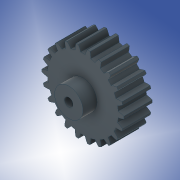
# Autodesk Inventor part: BA011
Saved by Autodesk Inventor 2017 (Build 210142000, 142)
## iProperties
Created: 2017-06-23
Part Number: BA011
Material: ABS Plastic
Document SubType Name: Modeling
Designer: zallen
Density: 1.06 g/cm^3
Appearance: CR Dark Blue
Author: zallen
Autodesk Inventor part; units mm, degrees
ref_plane "YZ Plane" through (0, 0, 0) normal (1, 0, 0) x (0, 1, 0)
ref_plane "XZ Plane" through (0, 0, 0) normal (0, 1, 0) x (-1, 0, 0)
ref_plane "XY Plane" through (0, 0, 0) normal (0, 0, 1) x (1, 0, 0)
sketch "Sketch1" plane through (0, 0, 0) normal (0, 0, 1) x (1, 0, 0)
  circle A0 centre (0, 0) radius 3
  circle A1 centre (0, 0) radius 25
  dimension "d0" = 6
  dimension "d1" = 50
  constraints: 2 centre point, 2 coincident
  measures "d0" diameter of A0
  measures "d1" diameter of A1
extrude "Extrusion1" add sketch "Sketch1" along normal blind 20
sketch "Sketch2" plane through (0, 0, 20) normal (0, 0, 1) x (1, 0, 0)
  line L0 (0, 0) -> (50, 0) construction
  circle A0 centre (0, 0) radius 25 projected
  circle A1 centre (0, 0) radius 25 projected
  arc A2 (28.9199, 0.9) -> (24.9199, 2) centre (22.9807, -12.8741) ccw
  arc A3 (28.9199, -0.9) -> (28.9199, 0.9) centre (8.9401, 0) ccw
  arc A4 (24.9199, -2) -> (28.9199, -0.9) centre (22.9807, 12.8741) ccw
  arc A5 (24.9199, -2) -> (24.9199, 2) centre (0, 0) ccw
  arc A6 (27.4949, 9.0112) -> (23.347, 8.9397) centre (25.6769, -5.8782) ccw
  arc A7 (28.002, 7.2841) -> (27.4949, 9.0112) centre (8.578, 2.5187) ccw
  arc A8 (24.4739, 5.1018) -> (28.002, 7.2841) centre (18.4228, 18.8271) ccw
  arc A9 (24.4739, 5.1018) -> (23.347, 8.9397) centre (0, 0) ccw
  arc A10 (23.8424, 16.3924) -> (19.8826, 15.1552) centre (26.2929, 1.5939) ccw
  arc A11 (24.8155, 14.8781) -> (23.8424, 16.3924) centre (7.5209, 4.8334) ccw
  arc A12 (22.0452, 11.7902) -> (24.8155, 14.8781) centre (12.3723, 23.2547) ccw
  arc A13 (22.0452, 11.7902) -> (19.8826, 15.1552) centre (0, 0) ccw
  arc A14 (18.2583, 22.4456) -> (14.8075, 20.1429) centre (24.7788, 8.9369) ccw
  arc A15 (19.6187, 21.2668) -> (18.2583, 22.4456) centre (5.8545, 6.7565) ccw
  arc A16 (17.8305, 17.5235) -> (19.6187, 21.2668) centre (5.3196, 25.7984) ccw
  arc A17 (17.8305, 17.5235) -> (14.8075, 20.1429) centre (0, 0) ccw
  arc A18 (11.1951, 26.6803) -> (8.5328, 23.4987) centre (21.2573, 15.5559) ccw
  arc A19 (12.8324, 25.9326) -> (11.1951, 26.6803) centre (3.7139, 8.1322) ccw
  arc A20 (12.1714, 21.8371) -> (12.8324, 25.9326) centre (-2.1642, 26.2521) ccw
  arc A21 (12.1714, 21.8371) -> (8.5328, 23.4987) centre (0, 0) ccw
  arc A22 (3.2249, 28.7536) -> (1.5668, 24.9509) centre (16.0136, 20.9146) ccw
  arc A23 (5.0066, 28.4974) -> (3.2249, 28.7536) centre (1.2723, 8.8491) ccw
  arc A24 (5.5261, 24.3816) -> (5.0066, 28.4974) centre (-9.4726, 24.579) ccw
  arc A25 (5.5261, 24.3816) -> (1.5668, 24.9509) centre (0, 0) ccw
  arc A26 (-5.0066, 28.4974) -> (-5.5261, 24.3816) centre (9.4726, 24.579) ccw
  arc A27 (-3.2249, 28.7536) -> (-5.0066, 28.4974) centre (-1.2723, 8.8491) ccw
  arc A28 (-1.5668, 24.9509) -> (-3.2249, 28.7536) centre (-16.0136, 20.9146) ccw
  arc A29 (-1.5668, 24.9509) -> (-5.5261, 24.3816) centre (0, 0) ccw
  arc A30 (-12.8324, 25.9326) -> (-12.1714, 21.8371) centre (2.1642, 26.2521) ccw
  arc A31 (-11.1951, 26.6803) -> (-12.8324, 25.9326) centre (-3.7139, 8.1322) ccw
  arc A32 (-8.5328, 23.4987) -> (-11.1951, 26.6803) centre (-21.2573, 15.5559) ccw
  arc A33 (-8.5328, 23.4987) -> (-12.1714, 21.8371) centre (0, 0) ccw
  arc A34 (-19.6187, 21.2668) -> (-17.8305, 17.5235) centre (-5.3196, 25.7984) ccw
  arc A35 (-18.2583, 22.4456) -> (-19.6187, 21.2668) centre (-5.8545, 6.7565) ccw
  arc A36 (-14.8075, 20.1429) -> (-18.2583, 22.4456) centre (-24.7788, 8.9369) ccw
  arc A37 (-14.8075, 20.1429) -> (-17.8305, 17.5235) centre (0, 0) ccw
  arc A38 (-24.8155, 14.8781) -> (-22.0452, 11.7902) centre (-12.3723, 23.2547) ccw
  arc A39 (-23.8424, 16.3924) -> (-24.8155, 14.8781) centre (-7.5209, 4.8334) ccw
  arc A40 (-19.8826, 15.1552) -> (-23.8424, 16.3924) centre (-26.2929, 1.5939) ccw
  arc A41 (-19.8826, 15.1552) -> (-22.0452, 11.7902) centre (0, 0) ccw
  arc A42 (-28.002, 7.2841) -> (-24.4739, 5.1018) centre (-18.4228, 18.8271) ccw
  arc A43 (-27.4949, 9.0112) -> (-28.002, 7.2841) centre (-8.578, 2.5187) ccw
  arc A44 (-23.347, 8.9397) -> (-27.4949, 9.0112) centre (-25.6769, -5.8782) ccw
  arc A45 (-23.347, 8.9397) -> (-24.4739, 5.1018) centre (0, 0) ccw
  arc A46 (-28.9199, -0.9) -> (-24.9199, -2) centre (-22.9807, 12.8741) ccw
  arc A47 (-28.9199, 0.9) -> (-28.9199, -0.9) centre (-8.9401, 0) ccw
  arc A48 (-24.9199, 2) -> (-28.9199, 0.9) centre (-22.9807, -12.8741) ccw
  arc A49 (-24.9199, 2) -> (-24.9199, -2) centre (0, 0) ccw
  arc A50 (-27.4949, -9.0112) -> (-23.347, -8.9397) centre (-25.6769, 5.8782) ccw
  arc A51 (-28.002, -7.2841) -> (-27.4949, -9.0112) centre (-8.578, -2.5187) ccw
  arc A52 (-24.4739, -5.1018) -> (-28.002, -7.2841) centre (-18.4228, -18.8271) ccw
  arc A53 (-24.4739, -5.1018) -> (-23.347, -8.9397) centre (0, 0) ccw
  arc A54 (-23.8424, -16.3924) -> (-19.8826, -15.1552) centre (-26.2929, -1.5939) ccw
  arc A55 (-24.8155, -14.8781) -> (-23.8424, -16.3924) centre (-7.5209, -4.8334) ccw
  arc A56 (-22.0452, -11.7902) -> (-24.8155, -14.8781) centre (-12.3723, -23.2547) ccw
  arc A57 (-22.0452, -11.7902) -> (-19.8826, -15.1552) centre (0, 0) ccw
  arc A58 (-18.2583, -22.4456) -> (-14.8075, -20.1429) centre (-24.7788, -8.9369) ccw
  arc A59 (-19.6187, -21.2668) -> (-18.2583, -22.4456) centre (-5.8545, -6.7565) ccw
  arc A60 (-17.8305, -17.5235) -> (-19.6187, -21.2668) centre (-5.3196, -25.7984) ccw
  arc A61 (-17.8305, -17.5235) -> (-14.8075, -20.1429) centre (0, 0) ccw
  arc A62 (-11.1951, -26.6803) -> (-8.5328, -23.4987) centre (-21.2573, -15.5559) ccw
  arc A63 (-12.8324, -25.9326) -> (-11.1951, -26.6803) centre (-3.7139, -8.1322) ccw
  arc A64 (-12.1714, -21.8371) -> (-12.8324, -25.9326) centre (2.1642, -26.2521) ccw
  arc A65 (-12.1714, -21.8371) -> (-8.5328, -23.4987) centre (0, 0) ccw
  arc A66 (-3.2249, -28.7536) -> (-1.5668, -24.9509) centre (-16.0136, -20.9146) ccw
  arc A67 (-5.0066, -28.4974) -> (-3.2249, -28.7536) centre (-1.2723, -8.8491) ccw
  arc A68 (-5.5261, -24.3816) -> (-5.0066, -28.4974) centre (9.4726, -24.579) ccw
  arc A69 (-5.5261, -24.3816) -> (-1.5668, -24.9509) centre (0, 0) ccw
  arc A70 (5.0066, -28.4974) -> (5.5261, -24.3816) centre (-9.4726, -24.579) ccw
  arc A71 (3.2249, -28.7536) -> (5.0066, -28.4974) centre (1.2723, -8.8491) ccw
  arc A72 (1.5668, -24.9509) -> (3.2249, -28.7536) centre (16.0136, -20.9146) ccw
  arc A73 (1.5668, -24.9509) -> (5.5261, -24.3816) centre (0, 0) ccw
  arc A74 (12.8324, -25.9326) -> (12.1714, -21.8371) centre (-2.1642, -26.2521) ccw
  arc A75 (11.1951, -26.6803) -> (12.8324, -25.9326) centre (3.7139, -8.1322) ccw
  arc A76 (8.5328, -23.4987) -> (11.1951, -26.6803) centre (21.2573, -15.5559) ccw
  arc A77 (8.5328, -23.4987) -> (12.1714, -21.8371) centre (0, 0) ccw
  arc A78 (19.6187, -21.2668) -> (17.8305, -17.5235) centre (5.3196, -25.7984) ccw
  arc A79 (18.2583, -22.4456) -> (19.6187, -21.2668) centre (5.8545, -6.7565) ccw
  arc A80 (14.8075, -20.1429) -> (18.2583, -22.4456) centre (24.7788, -8.9369) ccw
  arc A81 (14.8075, -20.1429) -> (17.8305, -17.5235) centre (0, 0) ccw
  arc A82 (24.8155, -14.8781) -> (22.0452, -11.7902) centre (12.3723, -23.2547) ccw
  arc A83 (23.8424, -16.3924) -> (24.8155, -14.8781) centre (7.5209, -4.8334) ccw
  arc A84 (19.8826, -15.1552) -> (23.8424, -16.3924) centre (26.2929, -1.5939) ccw
  arc A85 (19.8826, -15.1552) -> (22.0452, -11.7902) centre (0, 0) ccw
  arc A86 (28.002, -7.2841) -> (24.4739, -5.1018) centre (18.4228, -18.8271) ccw
  arc A87 (27.4949, -9.0112) -> (28.002, -7.2841) centre (8.578, -2.5187) ccw
  arc A88 (23.347, -8.9397) -> (27.4949, -9.0112) centre (25.6769, 5.8782) ccw
  arc A89 (23.347, -8.9397) -> (24.4739, -5.1018) centre (0, 0) ccw
  point P0 (28.9401, 0)
  point P1 (27.7679, 8.1534)
  point P2 (24.346, 15.6462)
  point P3 (18.9518, 21.8715)
  point P4 (12.0222, 26.3249)
  point P5 (4.1186, 28.6456)
  point P6 (-4.1186, 28.6456)
  point P7 (-12.0222, 26.3249)
  point P8 (-18.9518, 21.8715)
  point P9 (-24.346, 15.6462)
  point P10 (-27.7679, 8.1534)
  point P11 (-28.9401, 0)
  point P12 (-27.7679, -8.1534)
  point P13 (-24.346, -15.6462)
  point P14 (-18.9518, -21.8715)
  point P15 (-12.0222, -26.3249)
  point P16 (-4.1186, -28.6456)
  point P17 (4.1186, -28.6456)
  point P18 (12.0222, -26.3249)
  point P19 (18.9518, -21.8715)
  point P20 (24.346, -15.6462)
  point P21 (27.7679, -8.1534)
  dimension "d4" = 50
  dimension "d5" = 15
  dimension "d6" = 4
  dimension "d7" = 2
  dimension "d8" = 20
  dimension "d9" = 1.8
  dimension "d10" = 15
  dimension "d11" = 4
  dimension "d12" = 2
  dimension "d15" = 360
  constraints: 181 point on circle, 88 centre point, 3 coincident, 2 end point, 1 horizontal, 1 point on line, 285 other
  measures "d4" distance of L0.start L0.end
  measures "d5" radius of A2
  measures "d6" horizontal distance of A2.start A0.start
  measures "d7" distance from line of L0 A0.start
  measures "d8" radius of A3
  measures "d9" distance of A3.start A2.start
  measures "d10" radius of A4
  measures "d11" horizontal distance of A3.start A0.end
  measures "d12" distance from line of L0 A0.end
extrude "Extrusion2" add sketch "Sketch2" against normal blind 20 contours A0 A2 A3 A4 | A0 A6 A7 A8 | A86 A87 A88 A0 | A0 A10 A11 A12 | A82 A83 A84 A0 | A0 A14 A15 A16 | A78 A79 A80 A0 | A0 A18 A19 A20 | A74 A75 A76 A0 | A0 A22 A23 A24 | A70 A71 A72 A0 | A0 A26 A27 A28 | A66 A67 A68 A0 | A0 A30 A31 A32 | A62 A63 A64 A0 | A0 A34 A35 A36 | A58 A59 A60 A0 | A0 A38 A39 A40 | A54 A55 A56 A0 | A0 A42 A43 A44 | A50 A51 A52 A0 | A0 A46 A47 A48
sketch "Sketch3" plane through (0, 0, 20) normal (0, 0, 1) x (1, 0, 0)
  circle A0 centre (0, 0) radius 10
  circle A1 centre (0, 0) radius 3 projected
  dimension "d19" = 20
  constraints: 1 centre point, 1 coincident
  measures "d19" diameter of A0
extrude "Extrusion3" add sketch "Sketch3" along normal blind 10
body "Solid1"
